Autodesk Fusion 360 part; units mm, degrees
(part 2 of 5)
sketch "Sketch4" plane through (0, 0, 2) normal (0, 0, 1) x (1, 0, 0)
  arc A0 (-7.2751, -171.1221) -> (-4.8986, -171.1648) centre (-6.058, -169.5351) ccw
  arc A1 (4.8986, -171.1648) -> (-4.8986, -171.1648) centre (0, -178.05) ccw
  arc A2 (4.8986, -171.1648) -> (7.2751, -171.1221) centre (6.058, -169.5351) ccw
  line L0 (7.2751, -171.1221) -> (15.0344, -165.1715)
  arc A3 (15.0344, -165.1715) -> (16.0278, -163.817) centre (13.2088, -162.7909) ccw
  line L1 (16.0278, -163.817) -> (19.1143, -155.3371)
  arc A4 (19.1143, -155.3371) -> (19.6835, -152.7386) centre (9.7173, -151.9169) ccw
  line L2 (19.6835, -152.7386) -> (20.2399, -145.9914)
  arc A5 (20.2399, -145.9914) -> (20.25, -145.7449) centre (17.25, -145.7449) ccw
  line L3 (20.25, -145.7449) -> (20.25, -35.5)
  arc A6 (20.25, -35.5) -> (19.1875, -32.4184) centre (15.25, -35.5) ccw
  arc A7 (18.55, -30.5695) -> (19.1875, -32.4184) centre (21.55, -30.5695) ccw
  line L4 (18.55, -30.5695) -> (18.55, 0.8857)
  arc A8 (19, 2.4661) -> (18.55, 0.8857) centre (21.55, 0.8857) ccw
  arc A9 (19, 2.4661) -> (9.7944, 5.7648) centre (14.75, 5.1) ccw
  arc A10 (8.9423, 4.0423) -> (9.7944, 5.7648) centre (6.821, 6.1637) ccw
  line L5 (8.9423, 4.0423) -> (1.4142, -3.4858)
  arc A11 (-1.4142, -3.4858) -> (1.4142, -3.4858) centre (0, -2.0716) ccw
  line L6 (-1.4142, -3.4858) -> (-8.9423, 4.0423)
  arc A12 (-9.7944, 5.7648) -> (-8.9423, 4.0423) centre (-6.821, 6.1637) ccw
  arc A13 (-9.7944, 5.7648) -> (-19, 2.4661) centre (-14.75, 5.1) ccw
  arc A14 (-18.55, 0.8857) -> (-19, 2.4661) centre (-21.55, 0.8857) ccw
  line L7 (-18.55, 0.8857) -> (-18.55, -30.5695)
  arc A15 (-19.1875, -32.4184) -> (-18.55, -30.5695) centre (-21.55, -30.5695) ccw
  arc A16 (-19.1875, -32.4184) -> (-20.25, -35.5) centre (-15.25, -35.5) ccw
  line L8 (-20.25, -35.5) -> (-20.25, -145.7449)
  arc A17 (-20.25, -145.7449) -> (-20.2399, -145.9914) centre (-17.25, -145.7449) ccw
  line L9 (-20.2399, -145.9914) -> (-19.6835, -152.7386)
  arc A18 (-19.6835, -152.7386) -> (-19.1143, -155.3371) centre (-9.7173, -151.9169) ccw
  line L10 (-19.1143, -155.3371) -> (-16.0278, -163.817)
  arc A19 (-16.0278, -163.817) -> (-15.0344, -165.1715) centre (-13.2088, -162.7909) ccw
  line L11 (-15.0344, -165.1715) -> (-7.2751, -171.1221)
  arc A20 (4.253, -18.8853) -> (2.35, -19.8578) centre (3.55, -19.8578) ccw
  line L12 (4.253, -18.8853) -> (8.8217, -22.188)
  arc A21 (9.65, -23.8089) -> (8.8217, -22.188) centre (7.65, -23.8089) ccw
  line L13 (9.65, -23.8089) -> (9.65, -25.2396)
  arc A22 (6.43, -26.8244) -> (9.65, -25.2396) centre (7.65, -25.2396) ccw
  line L14 (6.43, -26.8244) -> (2.818, -24.044)
  arc A23 (2.35, -23.0931) -> (2.818, -24.044) centre (3.55, -23.0931) ccw
  line L15 (2.35, -23.0931) -> (2.35, -19.8578)
  circle A24 centre (11.5, -163.1) radius 1.5
  circle A25 centre (-15.25, -108.3) radius 1.5
  arc A26 (-11.75, -14.5) -> (-9.75, -14.5) centre (-10.75, -14.5) ccw
  line L16 (-11.75, -14.5) -> (-11.75, -2.5)
  arc A27 (-9.75, -2.5) -> (-11.75, -2.5) centre (-10.75, -2.5) ccw
  line L17 (-9.75, -2.5) -> (-9.75, -14.5)
  arc A28 (-13.55, -8.5) -> (-15.55, -8.5) centre (-14.55, -8.5) ccw
  line L18 (-13.55, -8.5) -> (-13.55, -20.5)
  arc A29 (-15.55, -20.5) -> (-13.55, -20.5) centre (-14.55, -20.5) ccw
  line L19 (-15.55, -20.5) -> (-15.55, -8.5)
  circle A30 centre (14.75, 5.1) radius 1.5
  circle A31 centre (15.25, -108.3) radius 1.5
  circle A32 centre (-14.75, 5.1) radius 1.5
  arc A33 (15.55, -8.5) -> (13.55, -8.5) centre (14.55, -8.5) ccw
  line L20 (15.55, -8.5) -> (15.55, -20.5)
  arc A34 (13.55, -20.5) -> (15.55, -20.5) centre (14.55, -20.5) ccw
  line L21 (13.55, -20.5) -> (13.55, -8.5)
  arc A35 (-9.65, -25.2396) -> (-6.43, -26.8244) centre (-7.65, -25.2396) ccw
  line L22 (-9.65, -25.2396) -> (-9.65, -23.8089)
  arc A36 (-8.8217, -22.188) -> (-9.65, -23.8089) centre (-7.65, -23.8089) ccw
  line L23 (-8.8217, -22.188) -> (-4.253, -18.8853)
  arc A37 (-2.35, -19.8578) -> (-4.253, -18.8853) centre (-3.55, -19.8578) ccw
  line L24 (-2.35, -19.8578) -> (-2.35, -23.0931)
  arc A38 (-2.818, -24.044) -> (-2.35, -23.0931) centre (-3.55, -23.0931) ccw
  line L25 (-2.818, -24.044) -> (-6.43, -26.8244)
  circle A39 centre (-15.25, -35.5) radius 1.5
  circle A40 centre (15.25, -35.5) radius 1.5
  circle A41 centre (-11.5, -163.1) radius 1.5
  arc A42 (11.75, -2.5) -> (9.75, -2.5) centre (10.75, -2.5) ccw
  line L26 (11.75, -2.5) -> (11.75, -14.5)
  arc A43 (9.75, -14.5) -> (11.75, -14.5) centre (10.75, -14.5) ccw
  line L27 (9.75, -14.5) -> (9.75, -2.5)
  line L28 (15.25, -35.5) -> (15.25, -108.3) construction
  line L29 (13.75, -41.5) -> (13.75, -66.5)
  arc A44 (13.75, -66.5) -> (16.75, -66.5) centre (15.25, -66.5) ccw
  line L30 (16.75, -66.5) -> (16.75, -41.5)
  arc A45 (16.75, -41.5) -> (13.75, -41.5) centre (15.25, -41.5) ccw
  line L31 (15.25, -40) -> (15.25, -68) construction
  line L32 (16.75, -102.3) -> (16.75, -77.3)
  arc A46 (16.75, -77.3) -> (13.75, -77.3) centre (15.25, -77.3) ccw
  line L33 (13.75, -77.3) -> (13.75, -102.3)
  arc A47 (13.75, -102.3) -> (16.75, -102.3) centre (15.25, -102.3) ccw
  line L34 (15.25, -103.8) -> (15.25, -75.8) construction
  line L35 (13.75, -114.3) -> (13.75, -139.3)
  arc A48 (13.75, -139.3) -> (16.75, -139.3) centre (15.25, -139.3) ccw
  line L36 (16.75, -139.3) -> (16.75, -114.3)
  arc A49 (16.75, -114.3) -> (13.75, -114.3) centre (15.25, -114.3) ccw
  line L37 (15.25, -112.8) -> (15.25, -140.8) construction
  line L38 (15.25, -114.3) -> (15.25, -108.3) construction
  line L39 (0, 1.75) -> (0, 22.5)
  arc A50 (-16.75, -66.5) -> (-13.75, -66.5) centre (-15.25, -66.5) ccw
  arc A51 (-13.75, -77.3) -> (-16.75, -77.3) centre (-15.25, -77.3) ccw
  line L40 (-15.25, -40) -> (-15.25, -68) construction
  line L41 (-16.75, -139.3) -> (-16.75, -114.3)
  arc A52 (-16.75, -102.3) -> (-13.75, -102.3) centre (-15.25, -102.3) ccw
  arc A53 (-16.75, -139.3) -> (-13.75, -139.3) centre (-15.25, -139.3) ccw
  line L42 (-16.75, -66.5) -> (-16.75, -41.5)
  arc A54 (-13.75, -114.3) -> (-16.75, -114.3) centre (-15.25, -114.3) ccw
  circle A55 centre (-15.25, -108.3) radius 1.5
  line L43 (-15.25, -103.8) -> (-15.25, -75.8) construction
  line L44 (-15.25, -112.8) -> (-15.25, -140.8) construction
  line L45 (-16.75, -102.3) -> (-16.75, -77.3)
  line L46 (-13.75, -114.3) -> (-13.75, -139.3)
  line L47 (-13.75, -77.3) -> (-13.75, -102.3)
  line L48 (-13.75, -41.5) -> (-13.75, -66.5)
  arc A56 (-13.75, -41.5) -> (-16.75, -41.5) centre (-15.25, -41.5) ccw
  line L49 (-15.25, -114.3) -> (-15.25, -108.3) construction
  point P0 (-15.25, -108.3)
  dimension "d23" = 3
  dimension "d24" = 4.5
  dimension "d25" = 28
  dimension "d26" = 3
  dimension "d27" = 4.5
  dimension "d28" = 28
  dimension "d29" = 3
  dimension "d30" = 4.5
  dimension "d31" = 28
  constraint coincident A6.centre A40.centre
  constraint coincident A31.centre L28.end
  constraint tangent L29 A44
  constraint tangent A44 L30
  constraint parallel L29 L30
  constraint tangent L30 A45
  constraint tangent L29 A45
  constraint midpoint A45 L31.start
  constraint midpoint A44 L31.end
  constraint coincident L28 L31.end
  constraint parallel L28 L31
  constraint tangent L32 A46
  constraint tangent A46 L33
  constraint parallel L32 L33
  constraint tangent L33 A47
  constraint tangent L32 A47
  constraint midpoint A47 L34.start
  constraint midpoint A46 L34.end
  constraint parallel L28 L34
  constraint coincident L28 L34.start
  constraint tangent L35 A48
  constraint tangent A48 L36
  constraint parallel L35 L36
  constraint tangent L36 A49
  constraint tangent L35 A49
  constraint midpoint A49 L37.start
  constraint midpoint A48 L37.end
  constraint parallel L28 L37
  constraint coincident A49.centre L38.start
  constraint parallel L28 L38
  constraint symmetric A31 L39 A55
  constraint symmetric A31.centre L39 P0
  constraint symmetric L29.start L39 L48.start
  constraint symmetric L29.end L39 A50.end
  constraint symmetric A44.end L39 A50.start
  constraint symmetric L30.end L39 L42.end
  constraint symmetric A44 L39 A50
  constraint symmetric A45 L39 A56
  constraint symmetric L31.start L39 L40.start
  constraint symmetric L31.end L39 L40.end
  constraint symmetric L32.start L39 A52.start
  constraint symmetric L32.end L39 A51.end
  constraint symmetric A46.end L39 A51.start
  constraint symmetric L33.end L39 A52.end
  constraint symmetric A46 L39 A51
  constraint symmetric A47 L39 A52
  constraint symmetric L34.start L39 L43.start
  constraint symmetric L34.end L39 L43.end
  constraint symmetric L35.start L39 A54.start
  constraint symmetric L35.end L39 A53.end
  constraint symmetric A48.end L39 L41.start
  constraint symmetric L36.end L39 L41.end
  constraint symmetric A48 L39 A53
  constraint symmetric A49 L39 A54
  constraint symmetric L37.start L39 L44.start
  constraint symmetric L37.end L39 L44.end
  constraint symmetric A49.centre L39 A54.centre
  measures "d23" diameter of A44
  measures "d24" distance of A6.centre L31.start
  measures "d25" distance of L31.start L31.end
  measures "d26" diameter of A46
  measures "d27" distance of A31.centre L34.start
  measures "d28" distance of L34.start L34.end
  measures "d29" diameter of A48
  measures "d30" distance of A31.centre L37.start
  measures "d31" distance of L37.start L37.end
extrude "Extrude2" cut sketch "Sketch4" against normal blind 2 contours L29 A44 L30 A45 | L32 A46 L33 A47 | L35 A48 L36 A49 | A50 L42 L48 A56 | A51 A52 L45 L47 | L41 A53 A54 L46
sketch "Sketch5" plane through (0, 0, 2) normal (0, 0, 1) x (1, 0, 0)
  line L0 (-13.75, -77.3) -> (-13.75, -102.3)
  arc A0 (-16.75, -102.3) -> (-13.75, -102.3) centre (-15.25, -102.3) ccw
  line L1 (-16.75, -102.3) -> (-16.75, -77.3)
  arc A1 (-13.75, -77.3) -> (-16.75, -77.3) centre (-15.25, -77.3) ccw
  line L2 (-13.75, -41.5) -> (-13.75, -66.5)
  arc A2 (-16.75, -66.5) -> (-13.75, -66.5) centre (-15.25, -66.5) ccw
  line L3 (-16.75, -66.5) -> (-16.75, -41.5)
  arc A3 (-13.75, -41.5) -> (-16.75, -41.5) centre (-15.25, -41.5) ccw
  line L4 (-13.75, -114.3) -> (-13.75, -139.3)
  arc A4 (-16.75, -139.3) -> (-13.75, -139.3) centre (-15.25, -139.3) ccw
  line L5 (-16.75, -139.3) -> (-16.75, -114.3)
  arc A5 (-13.75, -114.3) -> (-16.75, -114.3) centre (-15.25, -114.3) ccw
  line L6 (16.75, -77.3) -> (16.75, -102.3)
  arc A6 (13.75, -102.3) -> (16.75, -102.3) centre (15.25, -102.3) ccw
  line L7 (13.75, -102.3) -> (13.75, -77.3)
  arc A7 (16.75, -77.3) -> (13.75, -77.3) centre (15.25, -77.3) ccw
  line L8 (13.75, -66.5) -> (13.75, -41.5)
  arc A8 (16.75, -41.5) -> (13.75, -41.5) centre (15.25, -41.5) ccw
  line L9 (16.75, -41.5) -> (16.75, -66.5)
  arc A9 (13.75, -66.5) -> (16.75, -66.5) centre (15.25, -66.5) ccw
  line L10 (13.75, -139.3) -> (13.75, -114.3)
  arc A10 (16.75, -114.3) -> (13.75, -114.3) centre (15.25, -114.3) ccw
  line L11 (16.75, -114.3) -> (16.75, -139.3)
  arc A11 (13.75, -139.3) -> (16.75, -139.3) centre (15.25, -139.3) ccw
  arc A12 (-7.2751, -171.1221) -> (-4.8986, -171.1648) centre (-6.058, -169.5351) ccw
  arc A13 (4.8986, -171.1648) -> (-4.8986, -171.1648) centre (0, -178.05) ccw
  arc A14 (4.8986, -171.1648) -> (7.2751, -171.1221) centre (6.058, -169.5351) ccw
  line L12 (7.2751, -171.1221) -> (15.0344, -165.1715)
  arc A15 (15.0344, -165.1715) -> (16.0278, -163.817) centre (13.2088, -162.7909) ccw
  line L13 (16.0278, -163.817) -> (19.1143, -155.3371)
  arc A16 (19.1143, -155.3371) -> (19.6835, -152.7386) centre (9.7173, -151.9169) ccw
  line L14 (19.6835, -152.7386) -> (20.2399, -145.9914)
  arc A17 (20.2399, -145.9914) -> (20.25, -145.7449) centre (17.25, -145.7449) ccw
  line L15 (20.25, -145.7449) -> (20.25, -35.5)
  arc A18 (20.25, -35.5) -> (19.1875, -32.4184) centre (15.25, -35.5) ccw
  arc A19 (18.55, -30.5695) -> (19.1875, -32.4184) centre (21.55, -30.5695) ccw
  line L16 (18.55, -30.5695) -> (18.55, 0.8857)
  arc A20 (19, 2.4661) -> (18.55, 0.8857) centre (21.55, 0.8857) ccw
  arc A21 (19, 2.4661) -> (9.7944, 5.7648) centre (14.75, 5.1) ccw
  arc A22 (8.9423, 4.0423) -> (9.7944, 5.7648) centre (6.821, 6.1637) ccw
  line L17 (8.9423, 4.0423) -> (1.4142, -3.4858)
  arc A23 (-1.4142, -3.4858) -> (1.4142, -3.4858) centre (0, -2.0716) ccw
  line L18 (-1.4142, -3.4858) -> (-8.9423, 4.0423)
  arc A24 (-9.7944, 5.7648) -> (-8.9423, 4.0423) centre (-6.821, 6.1637) ccw
  arc A25 (-9.7944, 5.7648) -> (-19, 2.4661) centre (-14.75, 5.1) ccw
  arc A26 (-18.55, 0.8857) -> (-19, 2.4661) centre (-21.55, 0.8857) ccw
  line L19 (-18.55, 0.8857) -> (-18.55, -30.5695)
  arc A27 (-19.1875, -32.4184) -> (-18.55, -30.5695) centre (-21.55, -30.5695) ccw
  arc A28 (-19.1875, -32.4184) -> (-20.25, -35.5) centre (-15.25, -35.5) ccw
  line L20 (-20.25, -35.5) -> (-20.25, -145.7449)
  arc A29 (-20.25, -145.7449) -> (-20.2399, -145.9914) centre (-17.25, -145.7449) ccw
  line L21 (-20.2399, -145.9914) -> (-19.6835, -152.7386)
  arc A30 (-19.6835, -152.7386) -> (-19.1143, -155.3371) centre (-9.7173, -151.9169) ccw
  line L22 (-19.1143, -155.3371) -> (-16.0278, -163.817)
  arc A31 (-16.0278, -163.817) -> (-15.0344, -165.1715) centre (-13.2088, -162.7909) ccw
  line L23 (-15.0344, -165.1715) -> (-7.2751, -171.1221)
  arc A32 (4.253, -18.8853) -> (2.35, -19.8578) centre (3.55, -19.8578) ccw
  line L24 (4.253, -18.8853) -> (8.8217, -22.188)
  arc A33 (9.65, -23.8089) -> (8.8217, -22.188) centre (7.65, -23.8089) ccw
  line L25 (9.65, -23.8089) -> (9.65, -25.2396)
  arc A34 (6.43, -26.8244) -> (9.65, -25.2396) centre (7.65, -25.2396) ccw
  line L26 (6.43, -26.8244) -> (2.818, -24.044)
  arc A35 (2.35, -23.0931) -> (2.818, -24.044) centre (3.55, -23.0931) ccw
  line L27 (2.35, -23.0931) -> (2.35, -19.8578)
  circle A36 centre (11.5, -163.1) radius 1.5
  circle A37 centre (-15.25, -108.3) radius 1.5
  arc A38 (-11.75, -14.5) -> (-9.75, -14.5) centre (-10.75, -14.5) ccw
  line L28 (-11.75, -14.5) -> (-11.75, -2.5)
  arc A39 (-9.75, -2.5) -> (-11.75, -2.5) centre (-10.75, -2.5) ccw
  line L29 (-9.75, -2.5) -> (-9.75, -14.5)
  arc A40 (-13.55, -8.5) -> (-15.55, -8.5) centre (-14.55, -8.5) ccw
  line L30 (-13.55, -8.5) -> (-13.55, -20.5)
  arc A41 (-15.55, -20.5) -> (-13.55, -20.5) centre (-14.55, -20.5) ccw
  line L31 (-15.55, -20.5) -> (-15.55, -8.5)
  circle A42 centre (14.75, 5.1) radius 1.5
  circle A43 centre (15.25, -108.3) radius 1.5
  circle A44 centre (-14.75, 5.1) radius 1.5
  arc A45 (15.55, -8.5) -> (13.55, -8.5) centre (14.55, -8.5) ccw
  line L32 (15.55, -8.5) -> (15.55, -20.5)
  arc A46 (13.55, -20.5) -> (15.55, -20.5) centre (14.55, -20.5) ccw
  line L33 (13.55, -20.5) -> (13.55, -8.5)
  arc A47 (-9.65, -25.2396) -> (-6.43, -26.8244) centre (-7.65, -25.2396) ccw
  line L34 (-9.65, -25.2396) -> (-9.65, -23.8089)
  arc A48 (-8.8217, -22.188) -> (-9.65, -23.8089) centre (-7.65, -23.8089) ccw
  line L35 (-8.8217, -22.188) -> (-4.253, -18.8853)
  arc A49 (-2.35, -19.8578) -> (-4.253, -18.8853) centre (-3.55, -19.8578) ccw
  line L36 (-2.35, -19.8578) -> (-2.35, -23.0931)
  arc A50 (-2.818, -24.044) -> (-2.35, -23.0931) centre (-3.55, -23.0931) ccw
  line L37 (-2.818, -24.044) -> (-6.43, -26.8244)
  circle A51 centre (-15.25, -35.5) radius 1.5
  circle A52 centre (15.25, -35.5) radius 1.5
  circle A53 centre (-11.5, -163.1) radius 1.5
  arc A54 (11.75, -2.5) -> (9.75, -2.5) centre (10.75, -2.5) ccw
  line L38 (11.75, -2.5) -> (11.75, -14.5)
  arc A55 (9.75, -14.5) -> (11.75, -14.5) centre (10.75, -14.5) ccw
  line L39 (9.75, -14.5) -> (9.75, -2.5)
  line L40 (-8.75, -31.0716) -> (8.75, -31.0716)
  line L41 (8.75, -31.0716) -> (8.75, -44.0716)
  line L42 (0, -4.0716) -> (0, -169.6) construction
  line L43 (-8.75, -42.8216) -> (8.75, -42.8216)
  line L44 (-8.75, -31.0716) -> (-8.75, -44.0716)
  line L45 (0, -42.8216) -> (5, -42.8216)
  line L46 (8.75, -44.0716) -> (6.75, -44.0716)
  line L47 (6.75, -44.0716) -> (5, -42.8216)
  line L48 (0, -42.8216) -> (-5, -42.8216)
  line L49 (-8.75, -44.0716) -> (-6.75, -44.0716)
  line L50 (-6.75, -44.0716) -> (-5, -42.8216)
  line L51 (8.75, -31.0716) -> (5, -31.0716) construction
  line L52 (5, -31.0716) -> (5, -33.5716) construction
  line L53 (5, -33.5716) -> (8.75, -33.5716) construction
  line L54 (8.75, -33.5716) -> (8.75, -31.0716) construction
  line L55 (-8.75, -31.0716) -> (-5, -31.0716) construction
  line L56 (-5, -31.0716) -> (-5, -33.5716) construction
  line L57 (-5, -33.5716) -> (-8.75, -33.5716) construction
  line L58 (-8.75, -33.5716) -> (-8.75, -31.0716) construction
  line L59 (-8.75, -33.5716) -> (-5, -31.0716)
  line L60 (5, -31.0716) -> (8.75, -33.5716)
  line L61 (-5, -33.5716) -> (-5, -42.8216) construction
  line L62 (5, -33.5716) -> (5, -42.8216) construction
  point P0 (0, -4.0716)
  dimension "d34" = 27
  dimension "d35" = 8.75
  dimension "d36" = 17.5
  dimension "d37" = 13
  dimension "d38" = 11.75
  dimension "d39" = 13
  dimension "d40" = 5
  dimension "d41" = 2
  dimension "d42" = 5
  dimension "d43" = 2
  dimension "d45" = 2.5
  dimension "d47" = 2.5
  constraint horizontal L40
  constraint midpoint A23 P0
  constraint perpendicular L40 L41
  constraint coincident P0 L42.start
  constraint midpoint A13 L42.end
  constraint perpendicular L43 L44
  constraint midpoint L43 L45.start
  constraint perpendicular L42 L45
  constraint perpendicular L41 L46
  constraint perpendicular L42 L48
  constraint horizontal L49
  constraint horizontal L51
  constraint vertical L52
  constraint horizontal L53
  constraint vertical L54
  constraint horizontal L55
  constraint vertical L56
  constraint horizontal L57
  constraint vertical L58
  constraint vertical L61
  constraint vertical L62
  measures "d34" distance of L40 P0
  measures "d35" distance of L41 L42
  measures "d36" distance of L40.start L40.end
  measures "d37" distance of L40.end L41.end
  measures "d39" distance of L40.start L44.end
  measures "d40" distance of L45.start L45.end
  measures "d41" distance of L41.end L46.end
  measures "d42" distance of L45.start L48.end
  measures "d43" distance of L44.end L49.end
  measures "d45" distance of L40.end L53.end
  measures "d47" distance of L40.start L57.end
extrude "Extrude3" cut sketch "Sketch5" against normal blind 2 contours L40 L41 L43 L44 L45 L48 L59 L60 | L43 L44 L49 L50 | L41 L43 L46 L47
fillet "Fillet6" radius 1.5 6 edges at (8.75, -44.0716, 1) (6.75, -44.0716, 1) (-6.75, -44.0716, 1) (-8.75, -44.0716, 1) (-5, -42.8216, 1) (5, -42.8216, 1)
fillet "Fillet7" radius 3 4 edges at (-8.75, -33.5716, 1) (-5, -31.0716, 1) (5, -31.0716, 1) (8.75, -33.5716, 1)
sketch "Sketch6" plane through (0, 0, 2) normal (0, 0, 1) x (1, 0, 0)
  arc A0 (5.3912, -43.101) -> (4.5193, -42.8216) centre (4.5193, -44.3216) ccw
  line L0 (4.5193, -42.8216) -> (-4.5193, -42.8216)
  arc A1 (-4.5193, -42.8216) -> (-5.3912, -43.101) centre (-4.5193, -44.3216) ccw
  line L1 (-5.3912, -43.101) -> (-6.3588, -43.7922)
  arc A2 (-7.2307, -44.0716) -> (-6.3588, -43.7922) centre (-7.2307, -42.5716) ccw
  line L2 (-7.2307, -44.0716) -> (-7.25, -44.0716)
  arc A3 (-8.75, -42.5716) -> (-7.25, -44.0716) centre (-7.25, -42.5716) ccw
  line L3 (-8.75, -42.5716) -> (-8.75, -35.1771)
  arc A4 (-7.4141, -32.681) -> (-8.75, -35.1771) centre (-5.75, -35.1771) ccw
  line L4 (-7.4141, -32.681) -> (-5.7558, -31.5754)
  arc A5 (-4.0917, -31.0716) -> (-5.7558, -31.5754) centre (-4.0917, -34.0716) ccw
  line L5 (-4.0917, -31.0716) -> (4.0917, -31.0716)
  arc A6 (5.7558, -31.5754) -> (4.0917, -31.0716) centre (4.0917, -34.0716) ccw
  line L6 (5.7558, -31.5754) -> (7.4141, -32.681)
  arc A7 (8.75, -35.1771) -> (7.4141, -32.681) centre (5.75, -35.1771) ccw
  line L7 (8.75, -35.1771) -> (8.75, -42.5716)
  arc A8 (7.25, -44.0716) -> (8.75, -42.5716) centre (7.25, -42.5716) ccw
  line L8 (7.25, -44.0716) -> (7.2307, -44.0716)
  arc A9 (6.3588, -43.7922) -> (7.2307, -44.0716) centre (7.2307, -42.5716) ccw
  line L9 (6.3588, -43.7922) -> (5.3912, -43.101)
  line L10 (-13.75, -77.3) -> (-13.75, -102.3)
  arc A10 (-16.75, -102.3) -> (-13.75, -102.3) centre (-15.25, -102.3) ccw
  line L11 (-16.75, -102.3) -> (-16.75, -77.3)
  arc A11 (-13.75, -77.3) -> (-16.75, -77.3) centre (-15.25, -77.3) ccw
  line L12 (-13.75, -41.5) -> (-13.75, -66.5)
  arc A12 (-16.75, -66.5) -> (-13.75, -66.5) centre (-15.25, -66.5) ccw
  line L13 (-16.75, -66.5) -> (-16.75, -41.5)
  arc A13 (-13.75, -41.5) -> (-16.75, -41.5) centre (-15.25, -41.5) ccw
  line L14 (-13.75, -114.3) -> (-13.75, -139.3)
  arc A14 (-16.75, -139.3) -> (-13.75, -139.3) centre (-15.25, -139.3) ccw
  line L15 (-16.75, -139.3) -> (-16.75, -114.3)
  arc A15 (-13.75, -114.3) -> (-16.75, -114.3) centre (-15.25, -114.3) ccw
  line L16 (16.75, -77.3) -> (16.75, -102.3)
  arc A16 (13.75, -102.3) -> (16.75, -102.3) centre (15.25, -102.3) ccw
  line L17 (13.75, -102.3) -> (13.75, -77.3)
  arc A17 (16.75, -77.3) -> (13.75, -77.3) centre (15.25, -77.3) ccw
  line L18 (13.75, -66.5) -> (13.75, -41.5)
  arc A18 (16.75, -41.5) -> (13.75, -41.5) centre (15.25, -41.5) ccw
  line L19 (16.75, -41.5) -> (16.75, -66.5)
  arc A19 (13.75, -66.5) -> (16.75, -66.5) centre (15.25, -66.5) ccw
  line L20 (13.75, -139.3) -> (13.75, -114.3)
  arc A20 (16.75, -114.3) -> (13.75, -114.3) centre (15.25, -114.3) ccw
  line L21 (16.75, -114.3) -> (16.75, -139.3)
  arc A21 (13.75, -139.3) -> (16.75, -139.3) centre (15.25, -139.3) ccw
  arc A22 (-7.2751, -171.1221) -> (-4.8986, -171.1648) centre (-6.058, -169.5351) ccw
  arc A23 (4.8986, -171.1648) -> (-4.8986, -171.1648) centre (0, -178.05) ccw
  arc A24 (4.8986, -171.1648) -> (7.2751, -171.1221) centre (6.058, -169.5351) ccw
  line L22 (7.2751, -171.1221) -> (15.0344, -165.1715)
  arc A25 (15.0344, -165.1715) -> (16.0278, -163.817) centre (13.2088, -162.7909) ccw
  line L23 (16.0278, -163.817) -> (19.1143, -155.3371)
  arc A26 (19.1143, -155.3371) -> (19.6835, -152.7386) centre (9.7173, -151.9169) ccw
  line L24 (19.6835, -152.7386) -> (20.2399, -145.9914)
  arc A27 (20.2399, -145.9914) -> (20.25, -145.7449) centre (17.25, -145.7449) ccw
  line L25 (20.25, -145.7449) -> (20.25, -35.5)
  arc A28 (20.25, -35.5) -> (19.1875, -32.4184) centre (15.25, -35.5) ccw
  arc A29 (18.55, -30.5695) -> (19.1875, -32.4184) centre (21.55, -30.5695) ccw
  line L26 (18.55, -30.5695) -> (18.55, 0.8857)
  arc A30 (19, 2.4661) -> (18.55, 0.8857) centre (21.55, 0.8857) ccw
  arc A31 (19, 2.4661) -> (9.7944, 5.7648) centre (14.75, 5.1) ccw
  arc A32 (8.9423, 4.0423) -> (9.7944, 5.7648) centre (6.821, 6.1637) ccw
  line L27 (8.9423, 4.0423) -> (1.4142, -3.4858)
  arc A33 (-1.4142, -3.4858) -> (1.4142, -3.4858) centre (0, -2.0716) ccw
  line L28 (-1.4142, -3.4858) -> (-8.9423, 4.0423)
  arc A34 (-9.7944, 5.7648) -> (-8.9423, 4.0423) centre (-6.821, 6.1637) ccw
  arc A35 (-9.7944, 5.7648) -> (-19, 2.4661) centre (-14.75, 5.1) ccw
  arc A36 (-18.55, 0.8857) -> (-19, 2.4661) centre (-21.55, 0.8857) ccw
  line L29 (-18.55, 0.8857) -> (-18.55, -30.5695)
  arc A37 (-19.1875, -32.4184) -> (-18.55, -30.5695) centre (-21.55, -30.5695) ccw
  arc A38 (-19.1875, -32.4184) -> (-20.25, -35.5) centre (-15.25, -35.5) ccw
  line L30 (-20.25, -35.5) -> (-20.25, -145.7449)
  arc A39 (-20.25, -145.7449) -> (-20.2399, -145.9914) centre (-17.25, -145.7449) ccw
  line L31 (-20.2399, -145.9914) -> (-19.6835, -152.7386)
  arc A40 (-19.6835, -152.7386) -> (-19.1143, -155.3371) centre (-9.7173, -151.9169) ccw
  line L32 (-19.1143, -155.3371) -> (-16.0278, -163.817)
  arc A41 (-16.0278, -163.817) -> (-15.0344, -165.1715) centre (-13.2088, -162.7909) ccw
  line L33 (-15.0344, -165.1715) -> (-7.2751, -171.1221)
  arc A42 (4.253, -18.8853) -> (2.35, -19.8578) centre (3.55, -19.8578) ccw
  line L34 (4.253, -18.8853) -> (8.8217, -22.188)
  arc A43 (9.65, -23.8089) -> (8.8217, -22.188) centre (7.65, -23.8089) ccw
  line L35 (9.65, -23.8089) -> (9.65, -25.2396)
  arc A44 (6.43, -26.8244) -> (9.65, -25.2396) centre (7.65, -25.2396) ccw
  line L36 (6.43, -26.8244) -> (2.818, -24.044)
  arc A45 (2.35, -23.0931) -> (2.818, -24.044) centre (3.55, -23.0931) ccw
  line L37 (2.35, -23.0931) -> (2.35, -19.8578)
  circle A46 centre (11.5, -163.1) radius 1.5
  circle A47 centre (-15.25, -108.3) radius 1.5
  arc A48 (-11.75, -14.5) -> (-9.75, -14.5) centre (-10.75, -14.5) ccw
  line L38 (-11.75, -14.5) -> (-11.75, -2.5)
  arc A49 (-9.75, -2.5) -> (-11.75, -2.5) centre (-10.75, -2.5) ccw
  line L39 (-9.75, -2.5) -> (-9.75, -14.5)
  arc A50 (-13.55, -8.5) -> (-15.55, -8.5) centre (-14.55, -8.5) ccw
  line L40 (-13.55, -8.5) -> (-13.55, -20.5)
  arc A51 (-15.55, -20.5) -> (-13.55, -20.5) centre (-14.55, -20.5) ccw
  line L41 (-15.55, -20.5) -> (-15.55, -8.5)
  circle A52 centre (14.75, 5.1) radius 1.5
  circle A53 centre (15.25, -108.3) radius 1.5
  circle A54 centre (-14.75, 5.1) radius 1.5
  arc A55 (15.55, -8.5) -> (13.55, -8.5) centre (14.55, -8.5) ccw
  line L42 (15.55, -8.5) -> (15.55, -20.5)
  arc A56 (13.55, -20.5) -> (15.55, -20.5) centre (14.55, -20.5) ccw
  line L43 (13.55, -20.5) -> (13.55, -8.5)
  arc A57 (-9.65, -25.2396) -> (-6.43, -26.8244) centre (-7.65, -25.2396) ccw
  line L44 (-9.65, -25.2396) -> (-9.65, -23.8089)
  arc A58 (-8.8217, -22.188) -> (-9.65, -23.8089) centre (-7.65, -23.8089) ccw
  line L45 (-8.8217, -22.188) -> (-4.253, -18.8853)
  arc A59 (-2.35, -19.8578) -> (-4.253, -18.8853) centre (-3.55, -19.8578) ccw
  line L46 (-2.35, -19.8578) -> (-2.35, -23.0931)
  arc A60 (-2.818, -24.044) -> (-2.35, -23.0931) centre (-3.55, -23.0931) ccw
  line L47 (-2.818, -24.044) -> (-6.43, -26.8244)
  circle A61 centre (-15.25, -35.5) radius 1.5
  circle A62 centre (15.25, -35.5) radius 1.5
  circle A63 centre (-11.5, -163.1) radius 1.5
  arc A64 (11.75, -2.5) -> (9.75, -2.5) centre (10.75, -2.5) ccw
  line L48 (11.75, -2.5) -> (11.75, -14.5)
  arc A65 (9.75, -14.5) -> (11.75, -14.5) centre (10.75, -14.5) ccw
  line L49 (9.75, -14.5) -> (9.75, -2.5)
  line L50 (0, -42.8216) -> (0, -169.6) construction
  line L51 (2.4, -49.8216) -> (2.4, -59.8216)
  line L52 (9.8, -54.8129) -> (9.8, -65.6031)
  line L53 (2.4, -49.8216) -> (9.8, -54.8129)
  line L54 (2.4, -59.8216) -> (9.8, -65.6031)
  line L55 (2.4, -59.8216) -> (11.6334, -59.8216) construction
  dimension "d54" = 2.4
  dimension "d55" = 7.4
  dimension "d56" = 7
  dimension "d57" = 38
  dimension "d67" = 34
  dimension "d68" = 10
  constraint midpoint L0 L50.start
  constraint midpoint A23 L50.end
  constraint perpendicular L0 L51
  constraint parallel L51 L52
  constraint horizontal L55
  measures "d54" distance of L50 L51
  measures "d55" distance of L51 L52
  measures "d56" distance of L0 L51.start
  measures "d57" angle of L54 L55
  measures "d67" angle of L0 L53
  measures "d68" distance of L51.start L51.end
extrude "Extrude4" cut sketch "Sketch6" against normal blind 2 contours L51 L52 L53 L54
fillet "Fillet8" radius 1 1 edges at (2.4, -49.8216, 1)
fillet "Fillet9" radius 1.5 1 edges at (9.8, -65.6031, 1)
fillet "Fillet10" radius 1.5 2 edges at (9.8, -54.8129, 1) (2.4, -59.8216, 1)
pattern_linear "R-Pattern1" count 2 spacing 18 along (0, -1, 0) of "Extrude4", "Fillet8", "Fillet9", "Fillet10"
mirror "Mirror1" about plane through (0, 0, 0) normal (1, 0, 0) of "Extrude4", "Fillet8", "Fillet9", "Fillet10", "R-Pattern1"
sketch "Sketch8" plane through (0, 0, 2) normal (0, 0, 1) x (1, 0, 0)
  line L0 (-2.9765, -78.272) -> (-7.3765, -81.7096)
  arc A0 (-9.8, -80.5276) -> (-7.3765, -81.7096) centre (-8.3, -80.5276) ccw
  line L1 (-9.8, -80.5276) -> (-9.8, -73.6105)
  arc A1 (-9.1388, -72.3669) -> (-9.8, -73.6105) centre (-8.3, -73.6105) ccw
  line L2 (-9.1388, -72.3669) -> (-3.9592, -68.8733)
  arc A2 (-2.4, -69.7023) -> (-3.9592, -68.8733) centre (-3.4, -69.7023) ccw
  line L3 (-2.4, -69.7023) -> (-2.4, -77.09)
  arc A3 (-2.9765, -78.272) -> (-2.4, -77.09) centre (-3.9, -77.09) ccw
  line L4 (-2.9765, -60.272) -> (-7.3765, -63.7096)
  arc A4 (-9.8, -62.5276) -> (-7.3765, -63.7096) centre (-8.3, -62.5276) ccw
  line L5 (-9.8, -62.5276) -> (-9.8, -55.6105)
  arc A5 (-9.1388, -54.3669) -> (-9.8, -55.6105) centre (-8.3, -55.6105) ccw
  line L6 (-9.1388, -54.3669) -> (-3.9592, -50.8733)
  arc A6 (-2.4, -51.7023) -> (-3.9592, -50.8733) centre (-3.4, -51.7023) ccw
  line L7 (-2.4, -51.7023) -> (-2.4, -59.09)
  arc A7 (-2.9765, -60.272) -> (-2.4, -59.09) centre (-3.9, -59.09) ccw
  line L8 (7.3765, -81.7096) -> (2.9765, -78.272)
  arc A8 (2.4, -77.09) -> (2.9765, -78.272) centre (3.9, -77.09) ccw
  line L9 (2.4, -77.09) -> (2.4, -69.7023)
  arc A9 (3.9592, -68.8733) -> (2.4, -69.7023) centre (3.4, -69.7023) ccw
  line L10 (3.9592, -68.8733) -> (9.1388, -72.3669)
  arc A10 (9.8, -73.6105) -> (9.1388, -72.3669) centre (8.3, -73.6105) ccw
  line L11 (9.8, -73.6105) -> (9.8, -80.5276)
  arc A11 (7.3765, -81.7096) -> (9.8, -80.5276) centre (8.3, -80.5276) ccw
  line L12 (7.3765, -63.7096) -> (2.9765, -60.272)
  arc A12 (2.4, -59.09) -> (2.9765, -60.272) centre (3.9, -59.09) ccw
  line L13 (2.4, -59.09) -> (2.4, -51.7023)
  arc A13 (3.9592, -50.8733) -> (2.4, -51.7023) centre (3.4, -51.7023) ccw
  line L14 (3.9592, -50.8733) -> (9.1388, -54.3669)
  arc A14 (9.8, -55.6105) -> (9.1388, -54.3669) centre (8.3, -55.6105) ccw
  line L15 (9.8, -55.6105) -> (9.8, -62.5276)
  arc A15 (7.3765, -63.7096) -> (9.8, -62.5276) centre (8.3, -62.5276) ccw
  arc A16 (5.3912, -43.101) -> (4.5193, -42.8216) centre (4.5193, -44.3216) ccw
  line L16 (4.5193, -42.8216) -> (-4.5193, -42.8216)
  arc A17 (-4.5193, -42.8216) -> (-5.3912, -43.101) centre (-4.5193, -44.3216) ccw
  line L17 (-5.3912, -43.101) -> (-6.3588, -43.7922)
  arc A18 (-7.2307, -44.0716) -> (-6.3588, -43.7922) centre (-7.2307, -42.5716) ccw
  line L18 (-7.2307, -44.0716) -> (-7.25, -44.0716)
  arc A19 (-8.75, -42.5716) -> (-7.25, -44.0716) centre (-7.25, -42.5716) ccw
  line L19 (-8.75, -42.5716) -> (-8.75, -35.1771)
  arc A20 (-7.4141, -32.681) -> (-8.75, -35.1771) centre (-5.75, -35.1771) ccw
  line L20 (-7.4141, -32.681) -> (-5.7558, -31.5754)
  arc A21 (-4.0917, -31.0716) -> (-5.7558, -31.5754) centre (-4.0917, -34.0716) ccw
  line L21 (-4.0917, -31.0716) -> (4.0917, -31.0716)
  arc A22 (5.7558, -31.5754) -> (4.0917, -31.0716) centre (4.0917, -34.0716) ccw
  line L22 (5.7558, -31.5754) -> (7.4141, -32.681)
  arc A23 (8.75, -35.1771) -> (7.4141, -32.681) centre (5.75, -35.1771) ccw
  line L23 (8.75, -35.1771) -> (8.75, -42.5716)
  arc A24 (7.25, -44.0716) -> (8.75, -42.5716) centre (7.25, -42.5716) ccw
  line L24 (7.25, -44.0716) -> (7.2307, -44.0716)
  arc A25 (6.3588, -43.7922) -> (7.2307, -44.0716) centre (7.2307, -42.5716) ccw
  line L25 (6.3588, -43.7922) -> (5.3912, -43.101)
  line L26 (-13.75, -77.3) -> (-13.75, -102.3)
  arc A26 (-16.75, -102.3) -> (-13.75, -102.3) centre (-15.25, -102.3) ccw
  line L27 (-16.75, -102.3) -> (-16.75, -77.3)
  arc A27 (-13.75, -77.3) -> (-16.75, -77.3) centre (-15.25, -77.3) ccw
  line L28 (-13.75, -41.5) -> (-13.75, -66.5)
  arc A28 (-16.75, -66.5) -> (-13.75, -66.5) centre (-15.25, -66.5) ccw
  line L29 (-16.75, -66.5) -> (-16.75, -41.5)
  arc A29 (-13.75, -41.5) -> (-16.75, -41.5) centre (-15.25, -41.5) ccw
  line L30 (-13.75, -114.3) -> (-13.75, -139.3)
  arc A30 (-16.75, -139.3) -> (-13.75, -139.3) centre (-15.25, -139.3) ccw
  line L31 (-16.75, -139.3) -> (-16.75, -114.3)
  arc A31 (-13.75, -114.3) -> (-16.75, -114.3) centre (-15.25, -114.3) ccw
  line L32 (16.75, -77.3) -> (16.75, -102.3)
  arc A32 (13.75, -102.3) -> (16.75, -102.3) centre (15.25, -102.3) ccw
  line L33 (13.75, -102.3) -> (13.75, -77.3)
  arc A33 (16.75, -77.3) -> (13.75, -77.3) centre (15.25, -77.3) ccw
  line L34 (13.75, -66.5) -> (13.75, -41.5)
  arc A34 (16.75, -41.5) -> (13.75, -41.5) centre (15.25, -41.5) ccw
  line L35 (16.75, -41.5) -> (16.75, -66.5)
  arc A35 (13.75, -66.5) -> (16.75, -66.5) centre (15.25, -66.5) ccw
  line L36 (13.75, -139.3) -> (13.75, -114.3)
  arc A36 (16.75, -114.3) -> (13.75, -114.3) centre (15.25, -114.3) ccw
  line L37 (16.75, -114.3) -> (16.75, -139.3)
  arc A37 (13.75, -139.3) -> (16.75, -139.3) centre (15.25, -139.3) ccw
  arc A38 (-7.2751, -171.1221) -> (-4.8986, -171.1648) centre (-6.058, -169.5351) ccw
  arc A39 (4.8986, -171.1648) -> (-4.8986, -171.1648) centre (0, -178.05) ccw
  arc A40 (4.8986, -171.1648) -> (7.2751, -171.1221) centre (6.058, -169.5351) ccw
  line L38 (7.2751, -171.1221) -> (15.0344, -165.1715)
  arc A41 (15.0344, -165.1715) -> (16.0278, -163.817) centre (13.2088, -162.7909) ccw
  line L39 (16.0278, -163.817) -> (19.1143, -155.3371)
  arc A42 (19.1143, -155.3371) -> (19.6835, -152.7386) centre (9.7173, -151.9169) ccw
  line L40 (19.6835, -152.7386) -> (20.2399, -145.9914)
  arc A43 (20.2399, -145.9914) -> (20.25, -145.7449) centre (17.25, -145.7449) ccw
  line L41 (20.25, -145.7449) -> (20.25, -35.5)
  arc A44 (20.25, -35.5) -> (19.1875, -32.4184) centre (15.25, -35.5) ccw
  arc A45 (18.55, -30.5695) -> (19.1875, -32.4184) centre (21.55, -30.5695) ccw
  line L42 (18.55, -30.5695) -> (18.55, 0.8857)
  arc A46 (19, 2.4661) -> (18.55, 0.8857) centre (21.55, 0.8857) ccw
  arc A47 (19, 2.4661) -> (9.7944, 5.7648) centre (14.75, 5.1) ccw
  arc A48 (8.9423, 4.0423) -> (9.7944, 5.7648) centre (6.821, 6.1637) ccw
  line L43 (8.9423, 4.0423) -> (1.4142, -3.4858)
  arc A49 (-1.4142, -3.4858) -> (1.4142, -3.4858) centre (0, -2.0716) ccw
  line L44 (-1.4142, -3.4858) -> (-8.9423, 4.0423)
  arc A50 (-9.7944, 5.7648) -> (-8.9423, 4.0423) centre (-6.821, 6.1637) ccw
  arc A51 (-9.7944, 5.7648) -> (-19, 2.4661) centre (-14.75, 5.1) ccw
  arc A52 (-18.55, 0.8857) -> (-19, 2.4661) centre (-21.55, 0.8857) ccw
  line L45 (-18.55, 0.8857) -> (-18.55, -30.5695)
  arc A53 (-19.1875, -32.4184) -> (-18.55, -30.5695) centre (-21.55, -30.5695) ccw
  arc A54 (-19.1875, -32.4184) -> (-20.25, -35.5) centre (-15.25, -35.5) ccw
  line L46 (-20.25, -35.5) -> (-20.25, -145.7449)
  arc A55 (-20.25, -145.7449) -> (-20.2399, -145.9914) centre (-17.25, -145.7449) ccw
  line L47 (-20.2399, -145.9914) -> (-19.6835, -152.7386)
  arc A56 (-19.6835, -152.7386) -> (-19.1143, -155.3371) centre (-9.7173, -151.9169) ccw
  line L48 (-19.1143, -155.3371) -> (-16.0278, -163.817)
  arc A57 (-16.0278, -163.817) -> (-15.0344, -165.1715) centre (-13.2088, -162.7909) ccw
  line L49 (-15.0344, -165.1715) -> (-7.2751, -171.1221)
  arc A58 (4.253, -18.8853) -> (2.35, -19.8578) centre (3.55, -19.8578) ccw
  line L50 (4.253, -18.8853) -> (8.8217, -22.188)
  arc A59 (9.65, -23.8089) -> (8.8217, -22.188) centre (7.65, -23.8089) ccw
  line L51 (9.65, -23.8089) -> (9.65, -25.2396)
  arc A60 (6.43, -26.8244) -> (9.65, -25.2396) centre (7.65, -25.2396) ccw
  line L52 (6.43, -26.8244) -> (2.818, -24.044)
  arc A61 (2.35, -23.0931) -> (2.818, -24.044) centre (3.55, -23.0931) ccw
  line L53 (2.35, -23.0931) -> (2.35, -19.8578)
  circle A62 centre (11.5, -163.1) radius 1.5
  circle A63 centre (-15.25, -108.3) radius 1.5
  arc A64 (-11.75, -14.5) -> (-9.75, -14.5) centre (-10.75, -14.5) ccw
  line L54 (-11.75, -14.5) -> (-11.75, -2.5)
  arc A65 (-9.75, -2.5) -> (-11.75, -2.5) centre (-10.75, -2.5) ccw
  line L55 (-9.75, -2.5) -> (-9.75, -14.5)
  arc A66 (-13.55, -8.5) -> (-15.55, -8.5) centre (-14.55, -8.5) ccw
  line L56 (-13.55, -8.5) -> (-13.55, -20.5)
  arc A67 (-15.55, -20.5) -> (-13.55, -20.5) centre (-14.55, -20.5) ccw
  line L57 (-15.55, -20.5) -> (-15.55, -8.5)
  circle A68 centre (14.75, 5.1) radius 1.5
  circle A69 centre (15.25, -108.3) radius 1.5
  circle A70 centre (-14.75, 5.1) radius 1.5
  arc A71 (15.55, -8.5) -> (13.55, -8.5) centre (14.55, -8.5) ccw
  line L58 (15.55, -8.5) -> (15.55, -20.5)
  arc A72 (13.55, -20.5) -> (15.55, -20.5) centre (14.55, -20.5) ccw
  line L59 (13.55, -20.5) -> (13.55, -8.5)
  arc A73 (-9.65, -25.2396) -> (-6.43, -26.8244) centre (-7.65, -25.2396) ccw
  line L60 (-9.65, -25.2396) -> (-9.65, -23.8089)
  arc A74 (-8.8217, -22.188) -> (-9.65, -23.8089) centre (-7.65, -23.8089) ccw
  line L61 (-8.8217, -22.188) -> (-4.253, -18.8853)
  arc A75 (-2.35, -19.8578) -> (-4.253, -18.8853) centre (-3.55, -19.8578) ccw
  line L62 (-2.35, -19.8578) -> (-2.35, -23.0931)
  arc A76 (-2.818, -24.044) -> (-2.35, -23.0931) centre (-3.55, -23.0931) ccw
  line L63 (-2.818, -24.044) -> (-6.43, -26.8244)
  circle A77 centre (-15.25, -35.5) radius 1.5
  circle A78 centre (15.25, -35.5) radius 1.5
  circle A79 centre (-11.5, -163.1) radius 1.5
  arc A80 (11.75, -2.5) -> (9.75, -2.5) centre (10.75, -2.5) ccw
  line L64 (11.75, -2.5) -> (11.75, -14.5)
  arc A81 (9.75, -14.5) -> (11.75, -14.5) centre (10.75, -14.5) ccw
  line L65 (9.75, -14.5) -> (9.75, -2.5)
  line L66 (-13.75, -85.5776) -> (13.75, -85.5776) construction
  line L67 (8.3, -82.0276) -> (-8.3, -82.0276) construction
  line L68 (8.3, -89.1276) -> (-8.3, -89.1276) construction
  arc A82 (2.4, -101.453) -> (3.9592, -102.282) centre (3.4, -101.453) ccw
  arc A83 (-7.3765, -89.4456) -> (-9.8, -90.6276) centre (-8.3, -90.6276) ccw
  line L69 (-2.4, -101.453) -> (-2.4, -94.0653)
  arc A84 (-9.8, -97.5448) -> (-9.1388, -98.7883) centre (-8.3, -97.5448) ccw
  line L70 (3.9592, -102.282) -> (9.1388, -98.7883)
  arc A85 (2.9765, -92.8833) -> (2.4, -94.0653) centre (3.9, -94.0653) ccw
  arc A86 (9.1388, -98.7883) -> (9.8, -97.5448) centre (8.3, -97.5448) ccw
  line L71 (-2.9765, -92.8833) -> (-7.3765, -89.4456)
  arc A87 (-2.4, -94.0653) -> (-2.9765, -92.8833) centre (-3.9, -94.0653) ccw
  arc A88 (-3.9592, -102.282) -> (-2.4, -101.453) centre (-3.4, -101.453) ccw
  line L72 (7.3765, -89.4456) -> (2.9765, -92.8833)
  arc A89 (9.8, -90.6276) -> (7.3765, -89.4456) centre (8.3, -90.6276) ccw
  line L73 (2.4, -94.0653) -> (2.4, -101.453)
  line L74 (9.8, -97.5448) -> (9.8, -90.6276)
  line L75 (-9.1388, -98.7883) -> (-3.9592, -102.282)
  line L76 (-9.8, -90.6276) -> (-9.8, -97.5448)
  dimension "d75" = 3.55
  constraint coincident L26 L66.start
  constraint coincident L33 L66.end
  constraint perpendicular L33 L66
  constraint coincident A11 L67.start
  constraint coincident A0 L67.end
  constraint tangent A0 L67
  constraint tangent A11 L67
  constraint symmetric L0.start L66 L71.start
  constraint symmetric L0.end L66 A83.start
  constraint symmetric A0.start L66 A83.end
  constraint symmetric A0 L66 A83
  constraint symmetric L1.end L66 A84.start
  constraint symmetric A1.start L66 A84.end
  constraint symmetric A1 L66 A84
  constraint symmetric L2.end L66 A88.start
  constraint symmetric A2.start L66 L69.start
  constraint symmetric A2 L66 A88
  constraint symmetric L3.end L66 L69.end
  constraint symmetric A3 L66 A87
  constraint symmetric L8.start L66 L72.start
  constraint symmetric L8.end L66 A85.start
  constraint symmetric A8.start L66 A85.end
  constraint symmetric A8 L66 A85
  constraint symmetric L9.end L66 A82.start
  constraint symmetric A9.start L66 A82.end
  constraint symmetric A9 L66 A82
  constraint symmetric L10.end L66 L70.end
  constraint symmetric A10.start L66 A86.end
  constraint symmetric A10 L66 A86
  constraint symmetric L11.end L66 A89.start
  constraint symmetric A11 L66 A89
  constraint symmetric L66 L67.start L68.start
  constraint symmetric L66 L67.end L68.end
  measures "d75" distance of L66 L67
extrude "Extrude5" cut sketch "Sketch8" against normal blind 2 contours A82 L70 A85 A86 L72 A89 L73 L74 | A83 L69 A84 L71 A87 A88 L75 L76
pattern_linear "R-Pattern2" count 4 spacing 18 along (0, -1, 0) of "Extrude5"
equation "d35 = ( 17.5 / 2 ) * 1 mm"
equation "d54 = ( 4.8 / 2 ) * 1 mm"
equation "d75 = ( 7.1 / 2 ) * 1 mm"

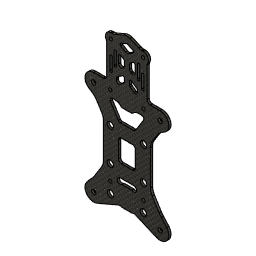
design "bottom_plate_2mm"
Autodesk Fusion 360 part; units mm, degrees